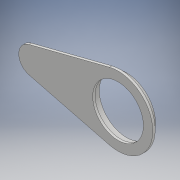
# Autodesk Inventor part: 101-bottom
Saved by Autodesk Inventor 2018 (Build 220112000, 112)
## iProperties
Created: 2019-11-07
Part Number: 101-bottom
Material: Generic
Document SubType Name: Modeling
Designer: Bunny320
Density: 1 g/cm^3
Appearance: Default
Author: Bunny320
Autodesk Inventor part; units mm, degrees
ref_plane "YZ Plane" through (0, 0, 0) normal (1, 0, 0) x (0, 1, 0)
ref_plane "XZ Plane" through (0, 0, 0) normal (0, 1, 0) x (-1, 0, 0)
ref_plane "XY Plane" through (0, 0, 0) normal (0, 0, 1) x (1, 0, 0)
sketch "Sketch2" plane through (0, 0, 0) normal (0, 1, 0) x (-1, 0, 0)
  circle A0 centre (0, 0) radius 22.5
  circle A1 centre (-141.8, 0) radius 57.5
  line L0 (5.5536, -21.8038) -> (-127.6075, -55.7209)
  line L1 (5.5536, 21.8038) -> (-127.6075, 55.7209)
  dimension "d5" = 141.8
  dimension "d6" = 45
  dimension "d7" = 115
  constraints: 4 end point, 4 point on circle, 4 tangent, 2 centre point, 1 coincident, 1 horizontal alignment
  measures "d5" distance of A1.centre point (0, 0)
  measures "d6" diameter of A0
  measures "d7" diameter of A1
extrude "Extrusion2" add sketch "Sketch2" along normal blind 4
sketch "Sketch5" plane through (0, 4, 0) normal (0, 1, 0) x (1, 0, 0)
  arc A0 (127.6075, -55.7209) -> (127.6075, 55.7209) centre (141.8, 0) ccw projected
  circle A1 centre (141.8, 0) radius 45
  circle A2 centre (141.8, 0) radius 48
  point P0 (0, 0)
  dimension "d17" = 90
  dimension "d18" = 96
  constraints: 2 centre point, 2 coincident
  measures "d17" diameter of A1
  measures "d18" diameter of A2
extrude "Extrusion5" add sketch "Sketch5" along normal blind 10
sketch "Sketch6" plane through (141.8, 4, 0) normal (0, 1, 0) x (1, 0, 0)
  arc A0 (-14.1925, -55.7209) -> (-14.1925, 55.7209) centre (0, 0) ccw projected
  circle A1 centre (0, 0) radius 42
  point P0 (-141.8, 0)
  dimension "d21" = 84
  constraints: 1 centre point, 1 coincident
  measures "d21" diameter of A1
extrude "Extrusion6" cut sketch "Sketch6" against normal through all
body "Solid2"
